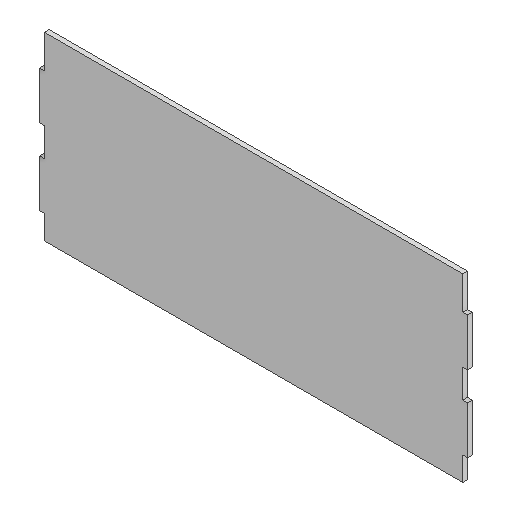
# Autodesk Inventor part: Piso
Saved by Autodesk Inventor 2022 (Build 260153000, 153)
## iProperties
Created: 2022-06-06
Part Number: Piso
Material: Generic
Document SubType Name: Modeling
Designer: ADMIN
Density: 1 g/cm^3
Appearance: Default
Author: ADMIN
Autodesk Inventor part; units mm, degrees
ref_plane "YZ Plane" through (0, 0, 0) normal (1, 0, 0) x (0, 1, 0)
ref_plane "XZ Plane" through (0, 0, 0) normal (0, 1, 0) x (-1, 0, 0)
ref_plane "XY Plane" through (0, 0, 0) normal (0, 0, 1) x (1, 0, 0)
sketch "Sketch1" plane through (0, 0, 0) normal (0, 0, 1) x (1, 0, 0)
  line L0 (505, 160) -> (505, 110) projected
  line L1 (505, 160) -> (500, 160) projected
  line L2 (500, 110) -> (500, 160) projected
  line L3 (505, 110) -> (500, 110) projected
  line L4 (505, 80) -> (505, 30) projected
  line L5 (505, 80) -> (500, 80) projected
  line L6 (500, 30) -> (500, 80) projected
  line L7 (505, 30) -> (500, 30) projected
  line L8 (60, 160) -> (60, 110) projected
  line L9 (60, 160) -> (55, 160) projected
  line L10 (55, 110) -> (55, 160) projected
  line L11 (60, 110) -> (55, 110) projected
  line L12 (60, 80) -> (60, 30) projected
  line L13 (60, 80) -> (55, 80) projected
  line L14 (55, 30) -> (55, 80) projected
  line L15 (60, 30) -> (55, 30) projected
  line L16 (55, 160) -> (60, 160) projected
  line L17 (60, 160) -> (60, 350) projected
  line L18 (60, 350) -> (55, 350) projected
  line L19 (55, 160) -> (55, 350) projected
  line L20 (60, 200) -> (500, 200) projected
  line L21 (500, 200) -> (500, 205) projected
  line L22 (60, 205) -> (500, 205) projected
  line L23 (500, 160) -> (505, 160) projected
  line L24 (505, 160) -> (505, 350) projected
  line L25 (505, 350) -> (500, 350) projected
  line L26 (500, 160) -> (500, 350) projected
  line L27 (505, 0) -> (500, 0) projected
  line L28 (500, 0) -> (500, -5) projected
  line L29 (505, -5) -> (500, -5) projected
  line L30 (505, 0) -> (505, -5) projected
  line L31 (60, 200) -> (500, 200)
  line L32 (500, 200) -> (500, 0)
  line L33 (500, 0) -> (60, 0)
  line L34 (60, 0) -> (60, 200)
  line L35 (500, 195) -> (60, 195)
  line L36 (60, 5) -> (500, 5)
  line L37 (60, 200) -> (60, 205) projected
  point P0 (0, 0)
  point P1 (60, 110)
  point P2 (60, 80)
  point P3 (60, 30)
  point P4 (60, 195)
  point P5 (50, 135)
  point P6 (55, 200)
  point P7 (60, 160)
  dimension "d2" = 5
  dimension "d3" = 5
  constraints: 12 end point, 4 point on line, 3 perpendicular, 2 parallel, 1 horizontal
  measures "d2" distance between parallel lines of L33 L36
  measures "d3" distance between parallel lines of L35 L31
extrude "Extrusion1" add sketch "Sketch1" along normal blind 5 contours L0 L3 L2 L1 | L2 L32 L6 L36 L34 L12 L8 L17 L35 L26 | L5 L4 L7 L6 | L8 L11 L10 L9 | L12 L15 L14 L13
body "Solid1"
